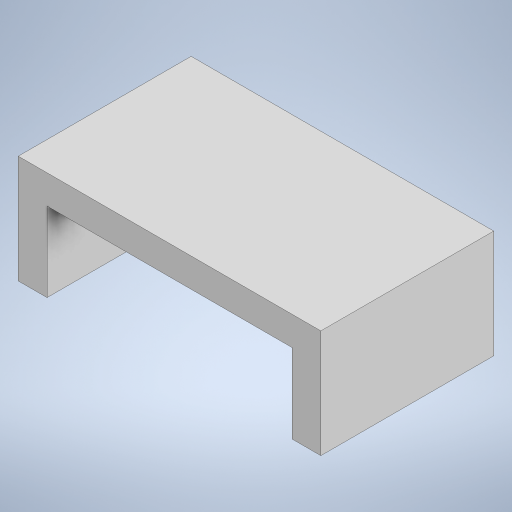
# Autodesk Inventor part: Table
Saved by Autodesk Inventor 2023 (Build 270158000, 158)
## iProperties
Created: 2022-11-15
Part Number: Table
Material: Generic
Document SubType Name: Modeling
Designer: Team 4026
Density: 1 g/cm^3
Appearance: Default
Author: Team 4026
Autodesk Inventor part; units mm, degrees
ref_plane "YZ Plane" through (0, 0, 0) normal (1, 0, 0) x (0, 1, 0)
ref_plane "XZ Plane" through (0, 0, 0) normal (0, 1, 0) x (-1, 0, 0)
ref_plane "XY Plane" through (0, 0, 0) normal (0, 0, 1) x (1, 0, 0)
sketch "Sketch2" plane through (0, 0, 0) normal (0, 1, 0) x (-1, 0, 0)
  line L0 (0, 0) -> (-2133.6, 0)
  line L1 (-2133.6, 0) -> (-2133.6, -1219.2)
  line L2 (-2133.6, -1219.2) -> (0, -1219.2)
  line L3 (0, -1219.2) -> (0, 0)
  dimension "d2" = 1219.2
  dimension "d3" = 2133.6
  constraints: 8 end point, 2 parallel, 1 horizontal, 1 perpendicular
  measures "d2" distance of L2.end L0.start
  measures "d3" distance of L0.start L0.end
extrude "Extrusion1" add sketch "Sketch2" along normal blind 762
shell "Shell1" thickness 203.2 removed faces 3 at (711.2, 508, 0) at (1422.4, 508, -1219.2) at (1422.4, 0, -406.4)
body "Solid1"
